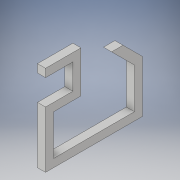
# Autodesk Inventor part: Main
Saved by Autodesk Inventor 2019 (Build 230136000, 136)
## iProperties
Created: 2018-08-02
Part Number: Main
Material: Generic
Document SubType Name: Modeling
Designer: zacha
Density: 1 g/cm^3
Appearance: Default
Author: zacha
Autodesk Inventor part; units mm, degrees
ref_plane "YZ Plane" through (0, 0, 0) normal (1, 0, 0) x (0, 1, 0)
ref_plane "XZ Plane" through (0, 0, 0) normal (0, 1, 0) x (-1, 0, 0)
ref_plane "XY Plane" through (0, 0, 0) normal (0, 0, 1) x (1, 0, 0)
sketch "Sketch1" plane through (0, 0, 0) normal (1, 0, 0) x (0, 1, 0)
  line L0 (0, 0) -> (20, 0) construction
  line L1 (20, 0) -> (20, -21.5)
  line L2 (20, -21.5) -> (0, -21.5)
  line L3 (0, -21.5) -> (0, 0)
  line L4 (20, 0) -> (26.35, 0)
  line L5 (26.35, 0) -> (26.35, -27.85)
  line L6 (-6.35, -27.85) -> (-6.35, -6.35)
  line L7 (-6.35, 0) -> (0, 0)
  line L8 (26.35, -27.85) -> (-6.35, -27.85)
  line L9 (-6.35, 0) -> (-44.45, 0)
  line L10 (-44.45, 0) -> (-44.45, -76.2)
  line L11 (-6.35, -6.35) -> (-38.1, -6.35)
  line L12 (-38.1, -6.35) -> (-38.1, -69.85)
  line L13 (-6.35, -6.35) -> (-6.35, 0) construction
  line L14 (-44.45, -76.2) -> (-3.7197, -76.2)
  line L15 (-38.1, -69.85) -> (-6.35, -69.85)
  line L16 (-6.35, -69.85) -> (11.6105, -51.8895)
  line L17 (-3.7197, -76.2) -> (11.6105, -60.8697)
  line L18 (11.6105, -51.8895) -> (11.6105, -60.8697)
  line L19 (-6.35, -27.85) -> (-6.35, -69.85) construction
  dimension "d0" = 20
  dimension "d1" = 21.5
  dimension "d2" = 6.35
  dimension "d4" = 6.35
  dimension "d23" = 6.35
  dimension "d24" = 38.1
  dimension "d25" = 76.2
  dimension "d26" = 6.35
  dimension "d27" = 6.35
  dimension "d28" = 6.35
  dimension "d30" = 6.35
  dimension "d31" = 25.4
  dimension "d32" = 135
  constraints: 40 end point, 7 perpendicular, 6 horizontal, 3 vertical, 2 parallel
  measures "d0" distance of L1.end L2.end
  measures "d1" distance of L0.end L1.end
  measures "d2" distance of L0.end L4.end
  measures "d4" distance between parallel lines of L6 L3
  measures "d23" distance between parallel lines of L2 L8
  measures "d24" distance of L7.start L9.end
  measures "d25" distance of L9.end L10.end
  measures "d26" distance between parallel lines of L9 L11
  measures "d27" distance between parallel lines of L10 L12
  measures "d28" distance between parallel lines of L14 L15
  measures "d30" distance between parallel lines of L17 L16
  measures "d31" distance of L15.end L16.end
  measures "d32" angle of L15 L16
extrude "Extrusion1" add sketch "Sketch1" along normal blind 6.35
body "Solid1"
